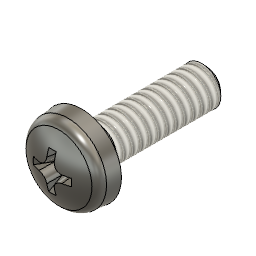
SLDP-71 (Autodesk Fusion 360 archive; units mm, degrees)
design "Pan Head Screw JIS B 1111 - M1.6 x 5 - H Steel 4.6 Plain"
description: Pan Head Screw JIS B 1111 - M1.6 x 5 - H
part number: PHS JIS B 1111 - M1.6 x 5 - H Steel 4.6 Plain
Autodesk Fusion 360 part; units mm, degrees
note: some values were not read from the file. Set by a fixed rule: which sketch regions a step uses.
sketch "Sketch1" plane through (0, 0, 0) normal (0, 1, 0) x (1, 0, 0)
  line L0 (-0.8, 0.7) -> (-0.8, 5)
  line L1 (-0.8, 5) -> (0, 5)
  line L2 (0, 5) -> (0, -1.3)
  line L3 (-0.6928, 0) -> (-1.6, 0)
  arc A0 (-1.5322, -0.7755) -> (0, -1.3) centre (0, 1.2) ccw
  line L4 (-0.8, 0.7) -> (-0.6928, 0.47)
  line L5 (-0.6928, 0.47) -> (-0.6928, 0)
  line L6 (-1.6, 0) -> (-1.5322, -0.7755)
  dimension "d9" = 1.6
  dimension "d66" = 3.2
  dimension "d75" = 1.3855
  dimension "d77" = 0.7
  dimension "d78" = 155
  dimension "d103" = 5
  dimension "d111" = 1.3
  dimension "d112" = 5
  constraint perpendicular L0 L1
  constraint collinear origin L2.end L1.end
  constraint perpendicular L0 L3
  constraint coincident origin L3
  constraint vertical L0
  constraint vertical L2
  constraint coincident L2 A0.centre
  constraint perpendicular L3 L5
  constraint coincident L3.start L5.end
  measures "d77" distance of L3 L0.start
  measures "d78" angle of L0 L4
  measures "d103" angle of L2 L6
  measures "d111" distance of L2.end L3
  measures "d112" distance of origin L1
revolve "Revolve1" add sketch "Sketch1" angle 360 about axis through (0, 0, -5) along (0, 0, 1) makes body 1
ref_plane "WorkPlane1" through (0, 0, 1.3) normal (0, 0, 1) x (1, 0, 0)
sketch "Sketch2" plane through (0, 0, 1.3) normal (0, 0, 1) x (1, 0, 0)
  line L0 (-0.155, 0.155) -> (-0.85, 0.155)
  line L1 (-0.155, -0.155) -> (-0.85, -0.155)
  line L2 (-0.85, 0.155) -> (-0.85, -0.155)
  line L3 (-0.155, -0.155) -> (-0.155, -0.85)
  line L4 (-0.155, -0.85) -> (0.155, -0.85)
  line L5 (0.155, -0.155) -> (0.155, -0.85)
  line L6 (0.155, -0.155) -> (0.85, -0.155)
  line L7 (0.85, -0.155) -> (0.85, 0.155)
  line L8 (0.155, 0.155) -> (0.85, 0.155)
  line L9 (0.155, 0.155) -> (0.155, 0.85)
  line L10 (0.155, 0.85) -> (-0.155, 0.85)
  line L11 (-0.155, 0.155) -> (-0.155, 0.85)
  dimension "d105" = 0.31
  dimension "d107" = 360
  dimension "d108" = 1.7
  constraint perpendicular L1 L2
  constraint vertical L0.start L1.start
  constraint horizontal L1
  constraint coincident L8.start L9.start
  measures "d105" distance of L0 L1
  measures "d108" distance of L2 L7
extrude "Extrude1" add sketch "Sketch2" against normal blind 0.95 draft -4 separate body makes body 2
draft "Draft1" angle -30 neutral plane through (0, 0, 1.3) pull (0, 0, 1) 4 faces at (-0.8279, 0.0295, 0.9833) (-0.0295, -0.8279, 0.9833) (0.8279, -0.0295, 0.9833) (0.0295, 0.8279, 0.9833) on bodies 2
fillet "Fillet3" radius 0.31 4 edges at (0.1218, 0.1218, 0.825) (-0.1218, 0.1218, 0.825) (0.1218, -0.1218, 0.825) (-0.1218, -0.1218, 0.825) on bodies 2
combine "Combine1" operation cut target body 1 tool bodies 2
fillet "Fillet4" radius 0.48 1 edges at (-1.4285, 0.5541, 0.7755) on bodies 1
thread "Thread1" "ISO Metric profile 1.6 M1.6x0.35 M1.6x0.35 6g" major diameter 1.5385 minor diameter 1.1385 pitch 0.35 angle 60 resizes the face on face at (-0.799, 0.0399, -3.5667) on bodies 1
fillet "Fillet5" radius 0.64 1 edges at (-0.6459, 0.2505, 0) on bodies 1
sketch "Sketch5" plane through (0, 0, 0) normal (0, 1, 0) x (1, 0, 0)
  line L0 (-0.816, 5) -> (-0.816, 4.7853)
  line L1 (-0.816, 4.7853) -> (-0.5853, 5)
  line L2 (0, 5) -> (0, -1.3)
  line L3 (-0.816, 5) -> (0, 5)
  dimension "d114" = 0.2147
  dimension "d115" = 0.816
  dimension "d116" = 0.2307
  constraint coincident L2.start L3.end
  constraint perpendicular L2 L3
  constraint coincident L1.end L3
  constraint perpendicular L0 L3
  measures "d114" distance of L0.end L3
  measures "d115" distance of L0 L2.start
  measures "d116" distance of L0 L1.end
revolve "Revolve2" cut sketch "Sketch5" angle 360 about axis through (0, 0, -5) along (0, 0, 1) bodies 1
equation "d9 = adsk_nomdia"
equation "adsk_nomlen = 5.00 mm"
equation "adsk_headh = 1.30 mm"
equation "adsk_headdia = 3.20 mm"
equation "adsk_nomdia = 1.60 mm"
equation "adsk_phildia = 1.70 mm"
equation "d31 = -adsk_phildepth"
equation "adsk_philwidth = 0.31 mm"
equation "adsk_phildepth = 0.95 mm"
equation "d66 = adsk_headdia"
equation "d71 = adsk_headh"
equation "adsk_thrlen = 4.30 mm"
equation "d75 = adsk_shnkdia"
equation "adsk_shnkdia = 1.3855 mm"
equation "d77 = adsk_nomlen - adsk_thrlen"
equation "adsk_endpointdia = 1.170585 mm"
equation "adsk_startlen = 0.2147075 mm"
equation "adsk_ovalrad = 2.50 mm"
equation "adsk_headtoprad = adsk_nomdia * 0.3"
equation "adsk_midfillet = 0.64 mm"
equation "d98 = adsk_midfillet"
equation "adsk_headang = 5.00 deg"
equation "d102 = adsk_headtoprad"
equation "d103 = adsk_headang"
equation "d105 = adsk_philwidth"
equation "d108 = adsk_phildia"
equation "d110 = adsk_philwidth"
equation "d111 = adsk_headh"
equation "d112 = adsk_nomlen"
equation "d113 = ( adsk_nomlen + adsk_headh ) - ( adsk_ovalrad )"
equation "d114 = adsk_startlen"
equation "d115 = adsk_nomdia * 0.51"
equation "d116 = ( adsk_nomdia * 0.51 ) - ( adsk_endpointdia / 2 )"

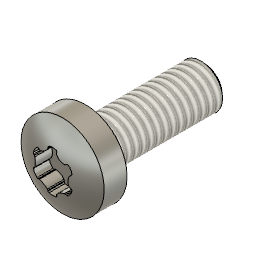
design "Hexalobular Socket Pan Head Screw SFS-EN ISO 14583 - M3x8 Stainless Steel A2 Plain"
description: Hexalobular Socket Pan Head Screw SFS-EN ISO 14583 - M3x8
part number: SFS-EN ISO 14583 - M3 x 8 Stainless Steel A2 Plain
Autodesk Fusion 360 part; units mm, degrees
sketch "Sketch1" plane through (0, 0, 0) normal (0, 1, 0) x (1, 0, 0)
  line L0 (-1.5, 8) -> (-1.5, 0)
  line L1 (-1.5, 0) -> (-2.8, 0)
  line L2 (-2.8, 0) -> (-2.8, -1.5425)
  arc A0 (-2.8, -1.5425) -> (0, -2.4) centre (0, 2.6) ccw
  line L3 (0, 8) -> (0, -2.4)
  line L4 (-1.5, 8) -> (0, 8)
  dimension "d128" = 5.6
  dimension "d129" = 3
  dimension "d167" = 2.4
  dimension "d168" = 8
  constraint perpendicular L0 L1
  constraint perpendicular L1 L2
  constraint vertical L3
  constraint coincident origin L3
  constraint coincident A0.centre L3
  constraint vertical L0
  constraint coincident origin L1
  constraint horizontal L4
  measures "d167" distance of L1 A0.end
  measures "d168" distance of L1 L4
revolve "Revolve1" add sketch "Sketch1" angle 360 about axis through (0, 0, -8) along (0, 0, 1)
ref_plane "WorkPlane2" through (0, 0, 2.4) normal (0, 0, 1) x (1, 0, 0)
sketch "Sketch2" plane through (0, 0, 2.4) normal (0, 0, 1) x (1, 0, 0)
  circle A0 centre (0, 0) radius 2.8
  line L0 (0, -2.8) -> (0, 2.8) construction
  circle A1 centre (0, 0) radius 1.092 construction
  circle A2 centre (0, 0) radius 1.379 construction
  circle A3 centre (0, 0) radius 1.4 construction
  line L1 (0, 0) -> (-0.2395, 1.358) construction
  line L2 (0, 0) -> (-0.2287, 1.3812) construction
  line L3 (0, 0) -> (-0.546, 0.9457)
  line L4 (0, 0) -> (-0.4035, 1.2202) construction
  arc A4 (0, 1.4) -> (-0.2395, 1.358) centre (0, 0.6956) ccw
  line L5 (0, 0.6956) -> (-0.2395, 1.358) construction
  circle A5 centre (-0.2125, 1.2833) radius 0.0794
  circle A6 centre (-0.9333, 1.6166) radius 0.7747
  line L6 (-0.9333, 1.6166) -> (-0.3131, 1.1525) construction
  circle A7 centre (-0.4035, 1.2202) radius 0.113
  line L7 (-0.2906, 1.2227) -> (-0.2919, 1.2816)
  arc A8 (0.2395, 1.358) -> (0, 1.4) centre (0, 0.6956) ccw
  circle A9 centre (0.2125, 1.2833) radius 0.0794
  line L8 (0.2906, 1.2227) -> (0.2919, 1.2816)
  circle A10 centre (0.4035, 1.2202) radius 0.113
  circle A11 centre (0.9333, 1.6166) radius 0.7747
  line L9 (0, 0) -> (0.546, 0.9457)
  line L10 (-0.9333, 1.6166) -> (-0.9333, 0) construction
  line L11 (-1.092, 0) -> (0, 0) construction
  line L12 (-0.9333, 1.6166) -> (0, 0) construction
  line L13 (-0.4035, 1.2202) -> (-0.4035, 0) construction
  point P0 (-0.2395, 1.358)
  point P1 (0, 1.4)
  point P2 (-0.2125, 1.2833)
  point P3 (-0.4035, 1.2202)
  dimension "d153" = 2.184
  dimension "d154" = 2.758
  dimension "d155" = 2.8
  dimension "d156" = 10
  dimension "d157" = 9.4
  dimension "d158" = 20
  dimension "d159" = 11.7
  dimension "d170" = 1.6166
  dimension "d171" = 1.2202
  constraint vertical L0
  constraint coincident A0 L0.end
  constraint coincident A0.centre L0
  constraint coincident A0 L0.start
  constraint concentric A0 A1
  constraint concentric A0 A2
  constraint concentric A2 A3
  constraint coincident A0.centre A1.centre
  constraint coincident A2 P0
  constraint coincident A3 L2.end
  constraint coincident A1 L3.end
  constraint coincident P0 L1.end
  constraint coincident L0 P1
  constraint coincident A3 P1
  constraint coincident P1 A4.start
  constraint coincident L0 A4.centre
  constraint coincident A4.centre L5.start
  constraint coincident L2 P2
  constraint coincident L5 P2
  constraint coincident P2 A5.centre
  constraint coincident P0 A5
  constraint coincident L3 A6.centre
  constraint coincident L3.end A6
  constraint coincident A6.centre L6.start
  constraint coincident A6 L6.end
  constraint coincident P3 L6
  constraint coincident P3 L4.end
  constraint coincident L6.end A7
  constraint coincident A7 L7.start
  constraint coincident A5 L7.end
  constraint tangent A5 L7
  constraint tangent A7 L7
  constraint symmetric L0 A0.centre A1.centre
  constraint symmetric L0 L3.end L9.end
  constraint symmetric L0 P1 A4.start
  constraint symmetric L0 P0 A8.start
  constraint symmetric L0 A4 A8
  constraint symmetric L0 A5 A9
  constraint symmetric L0 A6 A11
  constraint symmetric L0 A7 A10
  constraint symmetric L0 L7.start L8.start
  constraint symmetric L0 L7.end L8.end
  constraint vertical L10
  constraint perpendicular L10 L11
  constraint coincident A1 L11.start
  constraint coincident L10.end L11
  constraint coincident L11 L13.end
  constraint perpendicular L11 L13
  measures "d153" diameter of A1
  measures "d154" diameter of A2
  measures "d155" diameter of A3
  measures "d156" angle of L0 L1
  measures "d157" angle of L0 L2
  measures "d158" angle of L1 L3
  measures "d159" angle of L3 L4
  measures "d170" distance of A6.centre L11
  measures "d171" distance of P3 L11
extrude "Extrude6" cut sketch "Sketch2" against normal blind 1.27 contours L3 A4 A5 A6 A8 A9 A11 L9 | A9 L8 A10 A11 | A5 A6 A7 L7 | A4 A5 A6 | A5 A6 | A5 A6 | A8 A9 A11 | A9 A11 | A9 A11
pattern_circular "C-Pattern2" count 6 over 360 about axis through (0, 0, 1.75) along (0, 0, 1) of "Extrude6"
thread "Thread4" "ISO Metric profile 3.0 M3x0.5 M3x0.5 6g" major diameter 2.927 minor diameter 2.3555 pitch 0.5 angle 60 resizes the face on face at (-1.4925, 0.1494, -5.3333) from (0, 0, -1) to (0, 0, -8)
sketch "Sketch7" plane through (0, 0, 0) normal (0, 1, 0) x (1, 0, 0)
  line L0 (0, 8) -> (-1.53, 8)
  line L1 (-1.53, 7.7) -> (-1.2, 8)
  line L2 (-1.53, 7.7) -> (-1.53, 8)
  line L3 (0, 8) -> (0, -2.4)
  dimension "d172" = 1.53
  dimension "d173" = 0.3
  dimension "d174" = 0.33
  constraint coincident L1.end L0
  constraint coincident L0.start L3.start
  constraint perpendicular L0 L3
  constraint perpendicular L0 L2
  measures "d172" distance of L2 L0.start
  measures "d173" distance of L0 L1.start
  measures "d174" distance of L1.end L2
revolve "Revolve4" cut sketch "Sketch7" angle 360 about axis through (0, 0, 1.75) along (0, 0, 1)
equation "adsk_nomlen = 8.00 mm"
equation "adsk_headh = 2.40 mm"
equation "adsk_headdia = 5.60 mm"
equation "adsk_nomdia = 3.00 mm"
equation "adsk_phildia = 2.80 mm"
equation "adsk_phildepth = 1.27 mm"
equation "d125 = adsk_headh"
equation "d128 = adsk_headdia"
equation "d129 = adsk_nomdia"
equation "adsk_thrlen = 7.00 mm"
equation "adsk_startlen = 0.1 * adsk_nomdia"
equation "adsk_ovalrad = 5.00 mm"
equation "adsk_endpointdia = adsk_nomdia - adsk_startlen * 2"
equation "d153 = adsk_phildia * 0.78"
equation "d154 = adsk_phildia * 0.985"
equation "d155 = adsk_phildia"
equation "d162 = -adsk_phildepth"
equation "d167 = adsk_headh"
equation "d168 = adsk_nomlen"
equation "d169 = ( adsk_nomlen + adsk_headh ) - ( adsk_ovalrad )"
equation "d170 = ( adsk_phildia * 2 / 3 ) * sin(60 deg)"
equation "d171 = ( adsk_phildia * 0.459 ) * cos(18.3 deg)"
equation "d172 = adsk_nomdia * 0.51"
equation "d173 = adsk_startlen"
equation "d174 = ( adsk_nomdia * 0.51 ) - ( adsk_endpointdia / 2 )"
equation "d178 = min(adsk_thrlen; adsk_nomlen - 0.001 mm)"

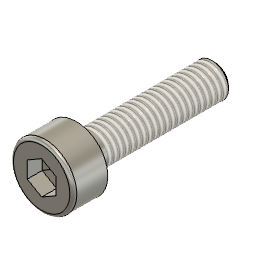
design "Hexagon Socket Head Cap Screw DIN EN ISO 4762 - M3 x 12 Stainless Steel A2 Plain"
description: Hexagon Socket Head Cap Screw DIN EN ISO 4762 - M3 x 12
part number: DIN EN ISO 4762 - M3 x 12 Stainless Steel A2 Plain
Autodesk Fusion 360 part; units mm, degrees
sketch "Sketch1" plane through (0, 0, 0) normal (0, 1, 0) x (1, 0, 0)
  line L0 (-1.5, 0) -> (-1.5, 12)
  line L1 (-1.5, 12) -> (0, 12)
  line L2 (0, 12) -> (0, -3)
  line L3 (-1.5, 0) -> (-2.75, 0)
  line L4 (-2.75, 0) -> (-2.75, -3)
  line L5 (-2.75, -3) -> (0, -3)
  dimension "d9" = 3
  dimension "d106" = 3
  dimension "d107" = 12
  dimension "d116" = 5.5
  constraint perpendicular L0 L1
  constraint collinear origin L1.end L2.end
  constraint perpendicular L0 L3
  constraint coincident origin L3
  constraint vertical L2
  constraint coincident L2 L5.end
  constraint perpendicular L2 L5
  measures "d106" distance of L3 L5
  measures "d107" distance of origin L1
revolve "Revolve1" add sketch "Sketch1" angle 360 about axis through (0, 0, -12) along (0, 0, 1)
ref_plane "WorkPlane1" through (0, 0, 3) normal (0, 0, 1) x (1, 0, 0)
sketch "Sketch6" plane through (0, 0, 3) normal (0, 0, 1) x (1, 0, 0)
  line L0 (-1.25, 0.7217) -> (-1.25, -0.7217)
  line L1 (-1.25, -0.7217) -> (0, -1.4434)
  line L2 (0, -1.4434) -> (1.25, -0.7217)
  line L3 (1.25, -0.7217) -> (1.25, 0.7217)
  line L4 (1.25, 0.7217) -> (0, 1.4434)
  line L5 (0, 1.4434) -> (-1.25, 0.7217)
  dimension "d117" = 2.5
  constraint vertical L0
  measures "d117" distance of L0 L3
extrude "Extrude1" cut sketch "Sketch6" against normal blind 1.3
extrude "Extrude2" cut 1 faces at (0, -0.4811, 1.7) along direction (0, 0, -1) blind 1.3 draft -85
fillet "Fillet4" radius 0.3 1 edges at (-2.5639, 0.9944, 3)
thread "Thread3" "ISO Metric profile 3.0 M3x0.5 M3x0.5 6g" major diameter 2.927 minor diameter 2.3555 pitch 0.5 angle 60 resizes the face on face at (-1.4981, 0.0748, -8) from (0, 0, -1.25) to (0, 0, -12)
sketch "Sketch7" plane through (0, 0, 0) normal (0, 1, 0) x (1, 0, 0)
  line L0 (-1.53, 12) -> (-1.53, 11.7)
  line L1 (-1.53, 11.7) -> (-1.23, 12)
  line L2 (0, 12) -> (0, -3)
  line L3 (-1.53, 12) -> (0, 12)
  dimension "d101" = 45
  dimension "d112" = 0.3
  dimension "d113" = 1.53
  constraint coincident L2.start L3.end
  constraint perpendicular L2 L3
  constraint coincident L1.end L3
  constraint perpendicular L0 L3
  measures "d101" angle of L0 L1
  measures "d112" distance of L0.end L3
  measures "d113" distance of L0 L2.start
revolve "Revolve3" cut sketch "Sketch7" angle 360 about axis through (0, 0, 1.75) along (0, 0, 1)
equation "d9 = adsk_nomdia"
equation "adsk_nomlen = 12.00 mm"
equation "adsk_headh = 3.00 mm"
equation "adsk_headdia = 5.50 mm"
equation "adsk_nomdia = 3.00 mm"
equation "adsk_philwidth = 2.50 mm"
equation "d31 = -adsk_phildepth"
equation "adsk_phildepth = 1.30 mm"
equation "d71 = adsk_headh"
equation "d76 = -adsk_phildepth"
equation "adsk_thrlen = 10.75 mm"
equation "d86 = adsk_nomdia * 0.1"
equation "adsk_startang = 45.00 deg"
equation "d101 = adsk_startang"
equation "adsk_pitch1 = 0.50 mm"
equation "adsk_startlen = 0.30 mm"
equation "d106 = adsk_headh"
equation "d107 = adsk_nomlen"
equation "d112 = adsk_startlen"
equation "d113 = adsk_nomdia * 0.51"
equation "d115 = min(adsk_thrlen; adsk_nomlen - 0.001 mm)"
equation "d116 = adsk_headdia"
equation "d117 = adsk_philwidth"

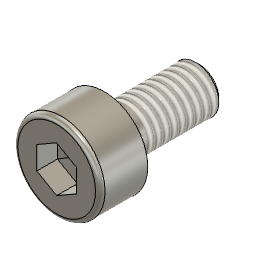
design "Hexagon Socket Head Cap Screw DIN EN ISO 4762 - M3 x 6 Stainless Steel A2 Plain"
description: Hexagon Socket Head Cap Screw DIN EN ISO 4762 - M3 x 6
part number: DIN EN ISO 4762 - M3 x 6 Stainless Steel A2 Plain
Autodesk Fusion 360 part; units mm, degrees
sketch "Sketch1" plane through (0, 0, 0) normal (0, 1, 0) x (1, 0, 0)
  line L0 (-1.5, 0) -> (-1.5, 6)
  line L1 (-1.5, 6) -> (0, 6)
  line L2 (0, 6) -> (0, -3)
  line L3 (-1.5, 0) -> (-2.75, 0)
  line L4 (-2.75, 0) -> (-2.75, -3)
  line L5 (-2.75, -3) -> (0, -3)
  dimension "d9" = 3
  dimension "d106" = 3
  dimension "d107" = 6
  dimension "d116" = 5.5
  constraint perpendicular L0 L1
  constraint collinear origin L1.end L2.end
  constraint perpendicular L0 L3
  constraint coincident origin L3
  constraint vertical L2
  constraint coincident L2 L5.end
  constraint perpendicular L2 L5
  measures "d106" distance of L3 L5
  measures "d107" distance of origin L1
revolve "Revolve1" add sketch "Sketch1" angle 360 about axis through (0, 0, -6) along (0, 0, 1)
ref_plane "WorkPlane1" through (0, 0, 3) normal (0, 0, 1) x (1, 0, 0)
sketch "Sketch6" plane through (0, 0, 3) normal (0, 0, 1) x (1, 0, 0)
  line L0 (-1.25, 0.7217) -> (-1.25, -0.7217)
  line L1 (-1.25, -0.7217) -> (0, -1.4434)
  line L2 (0, -1.4434) -> (1.25, -0.7217)
  line L3 (1.25, -0.7217) -> (1.25, 0.7217)
  line L4 (1.25, 0.7217) -> (0, 1.4434)
  line L5 (0, 1.4434) -> (-1.25, 0.7217)
  dimension "d117" = 2.5
  constraint vertical L0
  measures "d117" distance of L0 L3
extrude "Extrude1" cut sketch "Sketch6" against normal blind 1.3
extrude "Extrude2" cut 1 faces at (0, -0.4811, 1.7) along direction (0, 0, -1) blind 1.3 draft -85
fillet "Fillet4" radius 0.3 1 edges at (-2.5639, 0.9944, 3)
thread "Thread3" "ISO Metric profile 3.0 M3x0.5 M3x0.5 6g" major diameter 2.927 minor diameter 2.3555 pitch 0.5 angle 60 resizes the face on face at (-1.4925, 0.1494, -4) from (0, 0, -1.25) to (0, 0, -6)
sketch "Sketch7" plane through (0, 0, 0) normal (0, 1, 0) x (1, 0, 0)
  line L0 (-1.53, 6) -> (-1.53, 5.7)
  line L1 (-1.53, 5.7) -> (-1.23, 6)
  line L2 (0, 6) -> (0, -3)
  line L3 (-1.53, 6) -> (0, 6)
  dimension "d101" = 45
  dimension "d112" = 0.3
  dimension "d113" = 1.53
  constraint coincident L2.start L3.end
  constraint perpendicular L2 L3
  constraint coincident L1.end L3
  constraint perpendicular L0 L3
  measures "d101" angle of L0 L1
  measures "d112" distance of L0.end L3
  measures "d113" distance of L0 L2.start
revolve "Revolve3" cut sketch "Sketch7" angle 360 about axis through (0, 0, 1.75) along (0, 0, 1)
equation "d9 = adsk_nomdia"
equation "adsk_nomlen = 6.00 mm"
equation "adsk_headh = 3.00 mm"
equation "adsk_headdia = 5.50 mm"
equation "adsk_nomdia = 3.00 mm"
equation "adsk_philwidth = 2.50 mm"
equation "d31 = -adsk_phildepth"
equation "adsk_phildepth = 1.30 mm"
equation "d71 = adsk_headh"
equation "d76 = -adsk_phildepth"
equation "adsk_thrlen = 4.75 mm"
equation "d86 = adsk_nomdia * 0.1"
equation "adsk_startang = 45.00 deg"
equation "d101 = adsk_startang"
equation "adsk_pitch1 = 0.50 mm"
equation "adsk_startlen = 0.30 mm"
equation "d106 = adsk_headh"
equation "d107 = adsk_nomlen"
equation "d112 = adsk_startlen"
equation "d113 = adsk_nomdia * 0.51"
equation "d115 = min(adsk_thrlen; adsk_nomlen - 0.001 mm)"
equation "d116 = adsk_headdia"
equation "d117 = adsk_philwidth"

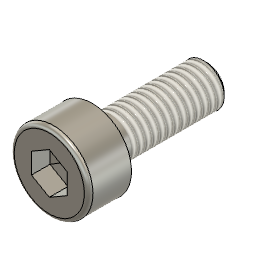
design "Hexagon Socket Head Cap Screw DIN EN ISO 4762 - M3 x 8 Stainless Steel A2 Plain"
description: Hexagon Socket Head Cap Screw DIN EN ISO 4762 - M3 x 8
part number: DIN EN ISO 4762 - M3 x 8 Stainless Steel A2 Plain
Autodesk Fusion 360 part; units mm, degrees
sketch "Sketch1" plane through (0, 0, 0) normal (0, 1, 0) x (1, 0, 0)
  line L0 (-1.5, 0) -> (-1.5, 8)
  line L1 (-1.5, 8) -> (0, 8)
  line L2 (0, 8) -> (0, -3)
  line L3 (-1.5, 0) -> (-2.75, 0)
  line L4 (-2.75, 0) -> (-2.75, -3)
  line L5 (-2.75, -3) -> (0, -3)
  dimension "d9" = 3
  dimension "d106" = 3
  dimension "d107" = 8
  dimension "d116" = 5.5
  constraint perpendicular L0 L1
  constraint collinear origin L1.end L2.end
  constraint perpendicular L0 L3
  constraint coincident origin L3
  constraint vertical L2
  constraint coincident L2 L5.end
  constraint perpendicular L2 L5
  measures "d106" distance of L3 L5
  measures "d107" distance of origin L1
revolve "Revolve1" add sketch "Sketch1" angle 360 about axis through (0, 0, -8) along (0, 0, 1)
ref_plane "WorkPlane1" through (0, 0, 3) normal (0, 0, 1) x (1, 0, 0)
sketch "Sketch6" plane through (0, 0, 3) normal (0, 0, 1) x (1, 0, 0)
  line L0 (-1.25, 0.7217) -> (-1.25, -0.7217)
  line L1 (-1.25, -0.7217) -> (0, -1.4434)
  line L2 (0, -1.4434) -> (1.25, -0.7217)
  line L3 (1.25, -0.7217) -> (1.25, 0.7217)
  line L4 (1.25, 0.7217) -> (0, 1.4434)
  line L5 (0, 1.4434) -> (-1.25, 0.7217)
  dimension "d117" = 2.5
  constraint vertical L0
  measures "d117" distance of L0 L3
extrude "Extrude1" cut sketch "Sketch6" against normal blind 1.3
extrude "Extrude2" cut 1 faces at (0, -0.4811, 1.7) along direction (0, 0, -1) blind 1.3 draft -85
fillet "Fillet4" radius 0.3 1 edges at (-2.5639, 0.9944, 3)
thread "Thread3" "ISO Metric profile 3.0 M3x0.5 M3x0.5 6g" major diameter 2.927 minor diameter 2.3555 pitch 0.5 angle 60 resizes the face on face at (-1.4925, 0.1494, -5.3333) from (0, 0, -1.25) to (0, 0, -8)
sketch "Sketch7" plane through (0, 0, 0) normal (0, 1, 0) x (1, 0, 0)
  line L0 (-1.53, 8) -> (-1.53, 7.7)
  line L1 (-1.53, 7.7) -> (-1.23, 8)
  line L2 (0, 8) -> (0, -3)
  line L3 (-1.53, 8) -> (0, 8)
  dimension "d101" = 45
  dimension "d112" = 0.3
  dimension "d113" = 1.53
  constraint coincident L2.start L3.end
  constraint perpendicular L2 L3
  constraint coincident L1.end L3
  constraint perpendicular L0 L3
  measures "d101" angle of L0 L1
  measures "d112" distance of L0.end L3
  measures "d113" distance of L0 L2.start
revolve "Revolve3" cut sketch "Sketch7" angle 360 about axis through (0, 0, 1.75) along (0, 0, 1)
equation "d9 = adsk_nomdia"
equation "adsk_nomlen = 8.00 mm"
equation "adsk_headh = 3.00 mm"
equation "adsk_headdia = 5.50 mm"
equation "adsk_nomdia = 3.00 mm"
equation "adsk_philwidth = 2.50 mm"
equation "d31 = -adsk_phildepth"
equation "adsk_phildepth = 1.30 mm"
equation "d71 = adsk_headh"
equation "d76 = -adsk_phildepth"
equation "adsk_thrlen = 6.75 mm"
equation "d86 = adsk_nomdia * 0.1"
equation "adsk_startang = 45.00 deg"
equation "d101 = adsk_startang"
equation "adsk_pitch1 = 0.50 mm"
equation "adsk_startlen = 0.30 mm"
equation "d106 = adsk_headh"
equation "d107 = adsk_nomlen"
equation "d112 = adsk_startlen"
equation "d113 = adsk_nomdia * 0.51"
equation "d115 = min(adsk_thrlen; adsk_nomlen - 0.001 mm)"
equation "d116 = adsk_headdia"
equation "d117 = adsk_philwidth"

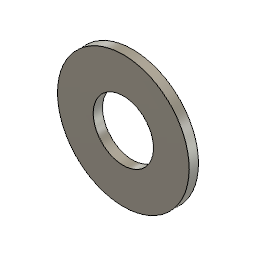
design "Washer DIN 125-1 - 3.2 - A Steel 100 HV Plain"
description: Washer DIN 125-1 - 3.2 - A
part number: DIN 125 - A 3.2 Steel 100 HV Plain
Autodesk Fusion 360 part; units mm, degrees
sketch "Sketch1" plane through (0, 0, 0) normal (0, 0, 1) x (1, 0, 0)
  circle A0 centre (0, 0) radius 3.5
  circle A1 centre (0, 0) radius 1.6
  dimension "d4" = 7
  dimension "d5" = 3.2
  constraint coincident A0.centre A1.centre
  measures "d4" diameter of A0
  measures "d5" diameter of A1
extrude "Extrude1" add sketch "Sketch1" along normal blind 0.5
equation "adsk_woutdia = 7.00 mm"
equation "adsk_windia = 3.20 mm"
equation "adsk_wthick = 0.50 mm"
equation "d4 = adsk_woutdia"
equation "d5 = adsk_windia"
equation "d6 = adsk_wthick"
equation "d30 = adsk_wthick"

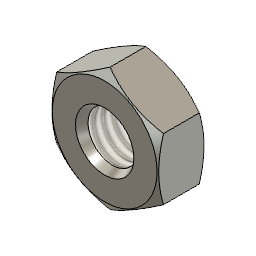
design "Hexagon Nut DIN 934 - M3 x 0.5 Stainless Steel A2 Plain"
description: Hexagon Nut DIN 934 - M3 x 0.5
part number: DIN 934 - M3 x 0.5 Stainless Steel A2 Plain
Autodesk Fusion 360 part; units mm, degrees
sketch "Sketch1" plane through (0, 0, 0) normal (0, 1, 0) x (1, 0, 0)
  line L0 (0, 0) -> (0, -2.4)
  line L1 (-1.5, 0) -> (-2.695, 0)
  line L2 (-2.695, 0) -> (-3.1763, -0.2778)
  line L3 (-3.1763, -0.2778) -> (-3.1763, -2.1222)
  line L4 (-3.1763, -2.1222) -> (-2.695, -2.4)
  line L5 (-2.695, -2.4) -> (-1.5, -2.4)
  line L6 (-1.5, -2.4) -> (-1.5, 0)
  dimension "d121" = 3
  dimension "d122" = 30
  dimension "d123" = 30
  dimension "d128" = 6.3525
  dimension "d172" = 5.39
  dimension "d179" = 2.4
  constraint vertical L0
  constraint coincident L0 L0.end
  constraint coincident origin L0
  constraint horizontal L1
  constraint coincident L0.start L1
  constraint coincident L0.start origin
  constraint coincident L0.end L5
  constraint vertical L1.end L4.end
  measures "d122" angle of L1 L2
  measures "d123" angle of L4 L5
  measures "d179" distance of L1 L5
revolve "Revolve1" add sketch "Sketch1" angle 360 about axis through (0, 0, 0) along (0, 0, 1)
sketch "Sketch8" plane through (0, 0, 2.4) normal (0, 0, 1) x (1, 0, 0)
  line L0 (-2.75, -1.5894) -> (-2.75, 1.5894)
  circle A0 centre (0, 0) radius 1.5
  circle A1 centre (0, 0) radius 3.1763
  dimension "d114" = 2.75
  constraint coincident L0.end A1
  constraint coincident L0.start A1
  constraint vertical L0
  measures "d114" distance of A0.centre L0
extrude "Extrude5" cut sketch "Sketch8" against normal blind 2.4 contours L0 A1 picked at (-2.8188, -0.3871)
pattern_circular "C-Pattern2" count 6 over 360 about axis through (0, 0, 1.75) along (0, 0, 1) of "Extrude5"
thread "Thread3" "ISO Metric profile 3.0 M3x0.5 M3x0.5 6H" major diameter 3.086 minor diameter 2.529 pitch 0.5 angle 60 resizes the face on face at (-1.4925, 0.1494, 1.6)
sketch "Sketch12" plane through (0, 0, 0) normal (0, 1, 0) x (1, 0, 0)
  line L0 (-1.5, 0) -> (0, 0)
  line L1 (-0.8072, -1.2) -> (-1.5, 0)
  line L2 (-1.5, -2.4) -> (0, -2.4)
  line L3 (-0.8072, -1.2) -> (-1.5, -2.4)
  line L4 (0, 0) -> (0, -2.4)
  dimension "d169" = 60
  dimension "d177" = 1.5
  dimension "d178" = 60
  constraint horizontal L0
  constraint coincident L1.start L3.start
  constraint vertical L0.start L2.start
  constraint coincident L2.end L4.end
  constraint coincident L0.end L4.start
  constraint perpendicular L2 L4
  measures "d169" angle of L2 L3
  measures "d177" distance of L0.start L4
  measures "d178" angle of L0 L1
revolve "Revolve3" cut sketch "Sketch12" angle 360 about axis through (0, 0, 1.75) along (0, 0, 1)
equation "adsk_nheig = 2.40 mm"
equation "adsk_maxdia = 6.3525 mm"
equation "adsk_nomdia = 3.00 mm"
equation "d89 = -adsk_nheig"
equation "adsk_waflat = 5.50 mm"
equation "d114 = adsk_waflat / 2"
equation "adsk_chamang1 = 30.00 deg"
equation "adsk_chamang2 = 30.00 deg"
equation "d121 = adsk_nomdia"
equation "d122 = adsk_chamang1"
equation "d123 = adsk_chamang2"
equation "d128 = adsk_maxdia"
equation "d163 = adsk_nheig"
equation "adsk_beardia = adsk_waflat * 0.98"
equation "d172 = adsk_beardia"
equation "d177 = adsk_nomdia * 0.5"
equation "d179 = adsk_nheig"

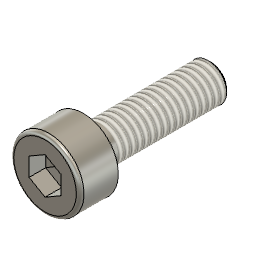
design "Hexagon Socket Head Cap Screw DIN EN ISO 4762 - M3 x 10 Stainless Steel A2 Plain"
description: Hexagon Socket Head Cap Screw DIN EN ISO 4762 - M3 x 10
part number: DIN EN ISO 4762 - M3 x 10 Stainless Steel A2 Plain
Autodesk Fusion 360 part; units mm, degrees
sketch "Sketch1" plane through (0, 0, 0) normal (0, 1, 0) x (1, 0, 0)
  line L0 (-1.5, 0) -> (-1.5, 10)
  line L1 (-1.5, 10) -> (0, 10)
  line L2 (0, 10) -> (0, -3)
  line L3 (-1.5, 0) -> (-2.75, 0)
  line L4 (-2.75, 0) -> (-2.75, -3)
  line L5 (-2.75, -3) -> (0, -3)
  dimension "d9" = 3
  dimension "d106" = 3
  dimension "d107" = 10
  dimension "d116" = 5.5
  constraint perpendicular L0 L1
  constraint collinear origin L1.end L2.end
  constraint perpendicular L0 L3
  constraint coincident origin L3
  constraint vertical L2
  constraint coincident L2 L5.end
  constraint perpendicular L2 L5
  measures "d106" distance of L3 L5
  measures "d107" distance of origin L1
revolve "Revolve1" add sketch "Sketch1" angle 360 about axis through (0, 0, -10) along (0, 0, 1)
ref_plane "WorkPlane1" through (0, 0, 3) normal (0, 0, 1) x (1, 0, 0)
sketch "Sketch6" plane through (0, 0, 3) normal (0, 0, 1) x (1, 0, 0)
  line L0 (-1.25, 0.7217) -> (-1.25, -0.7217)
  line L1 (-1.25, -0.7217) -> (0, -1.4434)
  line L2 (0, -1.4434) -> (1.25, -0.7217)
  line L3 (1.25, -0.7217) -> (1.25, 0.7217)
  line L4 (1.25, 0.7217) -> (0, 1.4434)
  line L5 (0, 1.4434) -> (-1.25, 0.7217)
  dimension "d117" = 2.5
  constraint vertical L0
  measures "d117" distance of L0 L3
extrude "Extrude1" cut sketch "Sketch6" against normal blind 1.3
extrude "Extrude2" cut 1 faces at (0, -0.4811, 1.7) along direction (0, 0, -1) blind 1.3 draft -85
fillet "Fillet4" radius 0.3 1 edges at (-2.5639, 0.9944, 3)
thread "Thread3" "ISO Metric profile 3.0 M3x0.5 M3x0.5 6g" major diameter 2.927 minor diameter 2.3555 pitch 0.5 angle 60 resizes the face on face at (-1.4925, 0.1494, -6.6667) from (0, 0, -1.25) to (0, 0, -10)
sketch "Sketch7" plane through (0, 0, 0) normal (0, 1, 0) x (1, 0, 0)
  line L0 (-1.53, 10) -> (-1.53, 9.7)
  line L1 (-1.53, 9.7) -> (-1.23, 10)
  line L2 (0, 10) -> (0, -3)
  line L3 (-1.53, 10) -> (0, 10)
  dimension "d101" = 45
  dimension "d112" = 0.3
  dimension "d113" = 1.53
  constraint coincident L2.start L3.end
  constraint perpendicular L2 L3
  constraint coincident L1.end L3
  constraint perpendicular L0 L3
  measures "d101" angle of L0 L1
  measures "d112" distance of L0.end L3
  measures "d113" distance of L0 L2.start
revolve "Revolve3" cut sketch "Sketch7" angle 360 about axis through (0, 0, 1.75) along (0, 0, 1)
equation "d9 = adsk_nomdia"
equation "adsk_nomlen = 10.00 mm"
equation "adsk_headh = 3.00 mm"
equation "adsk_headdia = 5.50 mm"
equation "adsk_nomdia = 3.00 mm"
equation "adsk_philwidth = 2.50 mm"
equation "d31 = -adsk_phildepth"
equation "adsk_phildepth = 1.30 mm"
equation "d71 = adsk_headh"
equation "d76 = -adsk_phildepth"
equation "adsk_thrlen = 8.75 mm"
equation "d86 = adsk_nomdia * 0.1"
equation "adsk_startang = 45.00 deg"
equation "d101 = adsk_startang"
equation "adsk_pitch1 = 0.50 mm"
equation "adsk_startlen = 0.30 mm"
equation "d106 = adsk_headh"
equation "d107 = adsk_nomlen"
equation "d112 = adsk_startlen"
equation "d113 = adsk_nomdia * 0.51"
equation "d115 = min(adsk_thrlen; adsk_nomlen - 0.001 mm)"
equation "d116 = adsk_headdia"
equation "d117 = adsk_philwidth"

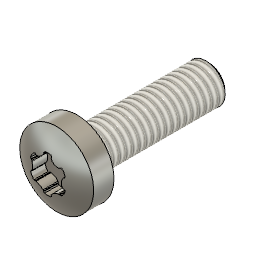
design "Hexalobular Socket Pan Head Screw SFS-EN ISO 14583 - M3x10 Stainless Steel A2 Plain"
description: Hexalobular Socket Pan Head Screw SFS-EN ISO 14583 - M3x10
part number: SFS-EN ISO 14583 - M3 x 10 Stainless Steel A2 Plain
Autodesk Fusion 360 part; units mm, degrees
sketch "Sketch1" plane through (0, 0, 0) normal (0, 1, 0) x (1, 0, 0)
  line L0 (-1.5, 10) -> (-1.5, 0)
  line L1 (-1.5, 0) -> (-2.8, 0)
  line L2 (-2.8, 0) -> (-2.8, -1.5425)
  arc A0 (-2.8, -1.5425) -> (0, -2.4) centre (0, 2.6) ccw
  line L3 (0, 10) -> (0, -2.4)
  line L4 (-1.5, 10) -> (0, 10)
  dimension "d128" = 5.6
  dimension "d129" = 3
  dimension "d167" = 2.4
  dimension "d168" = 10
  constraint perpendicular L0 L1
  constraint perpendicular L1 L2
  constraint vertical L3
  constraint coincident origin L3
  constraint coincident A0.centre L3
  constraint vertical L0
  constraint coincident origin L1
  constraint horizontal L4
  measures "d167" distance of L1 A0.end
  measures "d168" distance of L1 L4
revolve "Revolve1" add sketch "Sketch1" angle 360 about axis through (0, 0, -10) along (0, 0, 1)
ref_plane "WorkPlane2" through (0, 0, 2.4) normal (0, 0, 1) x (1, 0, 0)
sketch "Sketch2" plane through (0, 0, 2.4) normal (0, 0, 1) x (1, 0, 0)
  circle A0 centre (0, 0) radius 2.8
  line L0 (0, -2.8) -> (0, 2.8) construction
  circle A1 centre (0, 0) radius 1.092 construction
  circle A2 centre (0, 0) radius 1.379 construction
  circle A3 centre (0, 0) radius 1.4 construction
  line L1 (0, 0) -> (-0.2395, 1.358) construction
  line L2 (0, 0) -> (-0.2287, 1.3812) construction
  line L3 (0, 0) -> (-0.546, 0.9457)
  line L4 (0, 0) -> (-0.4035, 1.2202) construction
  arc A4 (0, 1.4) -> (-0.2395, 1.358) centre (0, 0.6956) ccw
  line L5 (0, 0.6956) -> (-0.2395, 1.358) construction
  circle A5 centre (-0.2125, 1.2833) radius 0.0794
  circle A6 centre (-0.9333, 1.6166) radius 0.7747
  line L6 (-0.9333, 1.6166) -> (-0.3131, 1.1525) construction
  circle A7 centre (-0.4035, 1.2202) radius 0.113
  line L7 (-0.2906, 1.2227) -> (-0.2919, 1.2816)
  arc A8 (0.2395, 1.358) -> (0, 1.4) centre (0, 0.6956) ccw
  circle A9 centre (0.2125, 1.2833) radius 0.0794
  line L8 (0.2906, 1.2227) -> (0.2919, 1.2816)
  circle A10 centre (0.4035, 1.2202) radius 0.113
  circle A11 centre (0.9333, 1.6166) radius 0.7747
  line L9 (0, 0) -> (0.546, 0.9457)
  line L10 (-0.9333, 1.6166) -> (-0.9333, 0) construction
  line L11 (-1.092, 0) -> (0, 0) construction
  line L12 (-0.9333, 1.6166) -> (0, 0) construction
  line L13 (-0.4035, 1.2202) -> (-0.4035, 0) construction
  point P0 (-0.2395, 1.358)
  point P1 (0, 1.4)
  point P2 (-0.2125, 1.2833)
  point P3 (-0.4035, 1.2202)
  dimension "d153" = 2.184
  dimension "d154" = 2.758
  dimension "d155" = 2.8
  dimension "d156" = 10
  dimension "d157" = 9.4
  dimension "d158" = 20
  dimension "d159" = 11.7
  dimension "d170" = 1.6166
  dimension "d171" = 1.2202
  constraint vertical L0
  constraint coincident A0 L0.end
  constraint coincident A0.centre L0
  constraint coincident A0 L0.start
  constraint concentric A0 A1
  constraint concentric A0 A2
  constraint concentric A2 A3
  constraint coincident A0.centre A1.centre
  constraint coincident A2 P0
  constraint coincident A3 L2.end
  constraint coincident A1 L3.end
  constraint coincident P0 L1.end
  constraint coincident L0 P1
  constraint coincident A3 P1
  constraint coincident P1 A4.start
  constraint coincident L0 A4.centre
  constraint coincident A4.centre L5.start
  constraint coincident L2 P2
  constraint coincident L5 P2
  constraint coincident P2 A5.centre
  constraint coincident P0 A5
  constraint coincident L3 A6.centre
  constraint coincident L3.end A6
  constraint coincident A6.centre L6.start
  constraint coincident A6 L6.end
  constraint coincident P3 L6
  constraint coincident P3 L4.end
  constraint coincident L6.end A7
  constraint coincident A7 L7.start
  constraint coincident A5 L7.end
  constraint tangent A5 L7
  constraint tangent A7 L7
  constraint symmetric L0 A0.centre A1.centre
  constraint symmetric L0 L3.end L9.end
  constraint symmetric L0 P1 A4.start
  constraint symmetric L0 P0 A8.start
  constraint symmetric L0 A4 A8
  constraint symmetric L0 A5 A9
  constraint symmetric L0 A6 A11
  constraint symmetric L0 A7 A10
  constraint symmetric L0 L7.start L8.start
  constraint symmetric L0 L7.end L8.end
  constraint vertical L10
  constraint perpendicular L10 L11
  constraint coincident A1 L11.start
  constraint coincident L10.end L11
  constraint coincident L11 L13.end
  constraint perpendicular L11 L13
  measures "d153" diameter of A1
  measures "d154" diameter of A2
  measures "d155" diameter of A3
  measures "d156" angle of L0 L1
  measures "d157" angle of L0 L2
  measures "d158" angle of L1 L3
  measures "d159" angle of L3 L4
  measures "d170" distance of A6.centre L11
  measures "d171" distance of P3 L11
extrude "Extrude6" cut sketch "Sketch2" against normal blind 1.27 contours L3 A4 A5 A6 A8 A9 A11 L9 | A9 L8 A10 A11 | A5 A6 A7 L7 | A4 A5 A6 | A5 A6 | A5 A6 | A8 A9 A11 | A9 A11 | A9 A11
pattern_circular "C-Pattern2" count 6 over 360 about axis through (0, 0, 1.75) along (0, 0, 1) of "Extrude6"
thread "Thread4" "ISO Metric profile 3.0 M3x0.5 M3x0.5 6g" major diameter 2.927 minor diameter 2.3555 pitch 0.5 angle 60 resizes the face on face at (-1.4925, 0.1494, -3.3333) from (0, 0, -1) to (0, 0, -10)
sketch "Sketch7" plane through (0, 0, 0) normal (0, 1, 0) x (1, 0, 0)
  line L0 (0, 10) -> (-1.53, 10)
  line L1 (-1.53, 9.7) -> (-1.2, 10)
  line L2 (-1.53, 9.7) -> (-1.53, 10)
  line L3 (0, 10) -> (0, -2.4)
  dimension "d172" = 1.53
  dimension "d173" = 0.3
  dimension "d174" = 0.33
  constraint coincident L1.end L0
  constraint coincident L0.start L3.start
  constraint perpendicular L0 L3
  constraint perpendicular L0 L2
  measures "d172" distance of L2 L0.start
  measures "d173" distance of L0 L1.start
  measures "d174" distance of L1.end L2
revolve "Revolve4" cut sketch "Sketch7" angle 360 about axis through (0, 0, 1.75) along (0, 0, 1)
equation "adsk_nomlen = 10.00 mm"
equation "adsk_headh = 2.40 mm"
equation "adsk_headdia = 5.60 mm"
equation "adsk_nomdia = 3.00 mm"
equation "adsk_phildia = 2.80 mm"
equation "adsk_phildepth = 1.27 mm"
equation "d125 = adsk_headh"
equation "d128 = adsk_headdia"
equation "d129 = adsk_nomdia"
equation "adsk_thrlen = 9.00 mm"
equation "adsk_startlen = 0.1 * adsk_nomdia"
equation "adsk_ovalrad = 5.00 mm"
equation "adsk_endpointdia = adsk_nomdia - adsk_startlen * 2"
equation "d153 = adsk_phildia * 0.78"
equation "d154 = adsk_phildia * 0.985"
equation "d155 = adsk_phildia"
equation "d162 = -adsk_phildepth"
equation "d167 = adsk_headh"
equation "d168 = adsk_nomlen"
equation "d169 = ( adsk_nomlen + adsk_headh ) - ( adsk_ovalrad )"
equation "d170 = ( adsk_phildia * 2 / 3 ) * sin(60 deg)"
equation "d171 = ( adsk_phildia * 0.459 ) * cos(18.3 deg)"
equation "d172 = adsk_nomdia * 0.51"
equation "d173 = adsk_startlen"
equation "d174 = ( adsk_nomdia * 0.51 ) - ( adsk_endpointdia / 2 )"
equation "d178 = min(adsk_thrlen; adsk_nomlen - 0.001 mm)"
